Autodesk Fusion 360 part; units mm, degrees
(part 5 of 5)
equation "d1182 = ( FootHeight ) + PanHeight - DeckThick"
equation "d1184 = ( BaseX + LeftRun + FaucetGap + RightRun - RightSideDepth ) + ( ( RightSideDepth ) - ( ( Wall + DeckClearance + RimBorder ) + ( ( RightSideDepth ) - 2 * ( Wall + DeckClearance + RimBorder ) ) ) )"
equation "d1185 = ( BaseY + Depth + ModuleGap ) + ( ( ( ( RightReach ) - ( 14 * SlotPitch + SlotWidth ) ) / 2 ) + ( 11 * SlotPitch ) )"
equation "d1186 = ( RightSideDepth ) - 2 * ( Wall + DeckClearance + RimBorder )"
equation "d1187 = SlotWidth"
equation "d1188 = DeckThick"
equation "d1190 = ( FootHeight ) + PanHeight - DeckThick"
equation "d1192 = ( BaseX + LeftRun + FaucetGap + RightRun - RightSideDepth ) + ( ( RightSideDepth ) - ( ( Wall + DeckClearance + RimBorder ) + ( ( RightSideDepth ) - 2 * ( Wall + DeckClearance + RimBorder ) ) ) )"
equation "d1193 = ( BaseY + Depth + ModuleGap ) + ( ( ( ( RightReach ) - ( 14 * SlotPitch + SlotWidth ) ) / 2 ) + ( 12 * SlotPitch ) )"
equation "d1194 = ( RightSideDepth ) - 2 * ( Wall + DeckClearance + RimBorder )"
equation "d1195 = SlotWidth"
equation "d1196 = DeckThick"
equation "d1198 = ( FootHeight ) + PanHeight - DeckThick"
equation "d1200 = ( BaseX + LeftRun + FaucetGap + RightRun - RightSideDepth ) + ( ( RightSideDepth ) - ( ( Wall + DeckClearance + RimBorder ) + ( ( RightSideDepth ) - 2 * ( Wall + DeckClearance + RimBorder ) ) ) )"
equation "d1201 = ( BaseY + Depth + ModuleGap ) + ( ( ( ( RightReach ) - ( 14 * SlotPitch + SlotWidth ) ) / 2 ) + ( 13 * SlotPitch ) )"
equation "d1202 = ( RightSideDepth ) - 2 * ( Wall + DeckClearance + RimBorder )"
equation "d1203 = SlotWidth"
equation "d1204 = DeckThick"
equation "d1206 = ( FootHeight ) + PanHeight - DeckThick"
equation "d1208 = ( BaseX + LeftRun + FaucetGap + RightRun - RightSideDepth ) + ( ( RightSideDepth ) - ( ( Wall + DeckClearance + RimBorder ) + ( ( RightSideDepth ) - 2 * ( Wall + DeckClearance + RimBorder ) ) ) )"
equation "d1209 = ( BaseY + Depth + ModuleGap ) + ( ( ( ( RightReach ) - ( 14 * SlotPitch + SlotWidth ) ) / 2 ) + ( 14 * SlotPitch ) )"
equation "d1210 = ( RightSideDepth ) - 2 * ( Wall + DeckClearance + RimBorder )"
equation "d1211 = SlotWidth"
equation "d1212 = DeckThick"
equation "d1214 = ( FootHeight ) + PanHeight - DeckThick"
equation "d1216 = ( BaseX + LeftRun + FaucetGap + RightRun - RightSideDepth ) + ( ( RightSideDepth ) - ( ( ( RightSideDepth ) - Wall - DeckClearance - 4 mm ) + ( 5 mm ) ) )"
equation "d1217 = ( BaseY + Depth + ModuleGap ) + ( ( RightReach ) / 2 - 8 mm )"
equation "d1220 = DeckThick"
equation "d1222 = TouchChamfer"
equation "d1223 = FootHeight + PanHeight - DeckThick"
equation "d1225 = ( BaseX ) + ( ( Wall ) - DeckClearance )"
equation "d1226 = ( BaseY ) + ( 10 mm - DeckClearance )"
equation "d1227 = 2 mm + 2 * DeckClearance"
equation "d1228 = 5 mm + 2 * DeckClearance"
equation "d1229 = DeckThick"
equation "d1231 = FootHeight"
equation "d1233 = ( BaseX ) + ( Wall )"
equation "d1234 = ( BaseY ) + ( 10 mm )"
equation "d1237 = PanHeight"
equation "d1239 = FootHeight + PanHeight - DeckThick"
equation "d1241 = ( BaseX ) + ( ( ( TowerWidth ) - Wall - 2 mm ) - DeckClearance )"
equation "d1242 = ( BaseY ) + ( 10 mm - DeckClearance )"
equation "d1243 = 2 mm + 2 * DeckClearance"
equation "d1244 = 5 mm + 2 * DeckClearance"
equation "d1245 = DeckThick"
equation "d1247 = FootHeight"
equation "d1249 = ( BaseX ) + ( ( TowerWidth ) - Wall - 2 mm )"
equation "d1250 = ( BaseY ) + ( 10 mm )"
equation "d1253 = PanHeight"
equation "d1255 = FootHeight + PanHeight - DeckThick"
equation "d1257 = ( BaseX + TowerWidth + ModuleGap ) + ( ( Wall ) - DeckClearance )"
equation "d1258 = ( BaseY ) + ( 10 mm - DeckClearance )"
equation "d1259 = 2 mm + 2 * DeckClearance"
equation "d1260 = 5 mm + 2 * DeckClearance"
equation "d1261 = DeckThick"
equation "d1263 = FootHeight"
equation "d1265 = ( BaseX + TowerWidth + ModuleGap ) + ( Wall )"
equation "d1266 = ( BaseY ) + ( 10 mm )"
equation "d1269 = PanHeight"
equation "d1271 = FootHeight + PanHeight - DeckThick"
equation "d1273 = ( BaseX + TowerWidth + ModuleGap ) + ( ( ( LeftRun - TowerWidth - ModuleGap ) - Wall - 2 mm ) - DeckClearance )"
equation "d1274 = ( BaseY ) + ( 10 mm - DeckClearance )"
equation "d1275 = 2 mm + 2 * DeckClearance"
equation "d1276 = 5 mm + 2 * DeckClearance"
equation "d1277 = DeckThick"
equation "d1279 = FootHeight"
equation "d1281 = ( BaseX + TowerWidth + ModuleGap ) + ( ( LeftRun - TowerWidth - ModuleGap ) - Wall - 2 mm )"
equation "d1282 = ( BaseY ) + ( 10 mm )"
equation "d1285 = PanHeight"
equation "d1287 = FootHeight + PanHeight - DeckThick"
equation "d1289 = ( BaseX + LeftRun + FaucetGap ) + ( ( Wall ) - DeckClearance )"
equation "d1290 = ( BaseY ) + ( 10 mm - DeckClearance )"
equation "d1291 = 2 mm + 2 * DeckClearance"
equation "d1292 = 5 mm + 2 * DeckClearance"
equation "d1293 = DeckThick"
equation "d1295 = FootHeight"
equation "d1297 = ( BaseX + LeftRun + FaucetGap ) + ( Wall )"
equation "d1298 = ( BaseY ) + ( 10 mm )"
equation "d1301 = PanHeight"
equation "d1303 = FootHeight + PanHeight - DeckThick"
equation "d1305 = ( BaseX + LeftRun + FaucetGap ) + ( ( ( ( RightRun - ModuleGap ) / 2 ) - Wall - 2 mm ) - DeckClearance )"
equation "d1306 = ( BaseY ) + ( 10 mm - DeckClearance )"
equation "d1307 = 2 mm + 2 * DeckClearance"
equation "d1308 = 5 mm + 2 * DeckClearance"
equation "d1309 = DeckThick"
equation "d1311 = FootHeight"
equation "d1313 = ( BaseX + LeftRun + FaucetGap ) + ( ( ( RightRun - ModuleGap ) / 2 ) - Wall - 2 mm )"
equation "d1314 = ( BaseY ) + ( 10 mm )"
equation "d1317 = PanHeight"
equation "d1319 = FootHeight + PanHeight - DeckThick"
equation "d1321 = ( BaseX + LeftRun + FaucetGap + ( RightRun + ModuleGap ) / 2 ) + ( ( Wall ) - DeckClearance )"
equation "d1322 = ( BaseY ) + ( 10 mm - DeckClearance )"
equation "d1323 = 2 mm + 2 * DeckClearance"
equation "d1324 = 5 mm + 2 * DeckClearance"
equation "d1325 = DeckThick"
equation "d1327 = FootHeight"
equation "d1329 = ( BaseX + LeftRun + FaucetGap + ( RightRun + ModuleGap ) / 2 ) + ( Wall )"
equation "d1330 = ( BaseY ) + ( 10 mm )"
equation "d1333 = PanHeight"
equation "d1335 = FootHeight + PanHeight - DeckThick"
equation "d1337 = ( BaseX + LeftRun + FaucetGap + ( RightRun + ModuleGap ) / 2 ) + ( ( ( ( RightRun - ModuleGap ) / 2 ) - Wall - 2 mm ) - DeckClearance )"
equation "d1338 = ( BaseY ) + ( 10 mm - DeckClearance )"
equation "d1339 = 2 mm + 2 * DeckClearance"
equation "d1340 = 5 mm + 2 * DeckClearance"
equation "d1341 = DeckThick"
equation "d1343 = FootHeight"
equation "d1345 = ( BaseX + LeftRun + FaucetGap + ( RightRun + ModuleGap ) / 2 ) + ( ( ( RightRun - ModuleGap ) / 2 ) - Wall - 2 mm )"
equation "d1346 = ( BaseY ) + ( 10 mm )"
equation "d1349 = PanHeight"
equation "d1351 = FootHeight + PanHeight - DeckThick"
equation "d1353 = ( BaseX ) + ( 10 mm - DeckClearance )"
equation "d1354 = ( BaseY + Depth + ModuleGap ) + ( ( LeftReach ) - ( ( ( Wall ) - DeckClearance ) + ( 2 mm + 2 * DeckClearance ) ) )"
equation "d1355 = 5 mm + 2 * DeckClearance"
equation "d1356 = 2 mm + 2 * DeckClearance"
equation "d1357 = DeckThick"
equation "d1359 = FootHeight"
equation "d1361 = ( BaseX ) + ( 10 mm )"
equation "d1362 = ( BaseY + Depth + ModuleGap ) + ( ( LeftReach ) - ( ( Wall ) + ( 2 mm ) ) )"
equation "d1365 = PanHeight"
equation "d1367 = FootHeight + PanHeight - DeckThick"
equation "d1369 = ( BaseX ) + ( 10 mm - DeckClearance )"
equation "d1370 = ( BaseY + Depth + ModuleGap ) + ( ( LeftReach ) - ( ( ( ( LeftReach ) - Wall - 2 mm ) - DeckClearance ) + ( 2 mm + 2 * DeckClearance ) ) )"
equation "d1371 = 5 mm + 2 * DeckClearance"
equation "d1372 = 2 mm + 2 * DeckClearance"
equation "d1373 = DeckThick"
equation "d1375 = FootHeight"
equation "d1377 = ( BaseX ) + ( 10 mm )"
equation "d1378 = ( BaseY + Depth + ModuleGap ) + ( ( LeftReach ) - ( ( ( LeftReach ) - Wall - 2 mm ) + ( 2 mm ) ) )"
equation "d1381 = PanHeight"
equation "d1383 = FootHeight + PanHeight - DeckThick"
equation "d1385 = ( BaseX + LeftRun + FaucetGap + RightRun - RightSideDepth ) + ( ( RightSideDepth ) - ( ( 10 mm - DeckClearance ) + ( 5 mm + 2 * DeckClearance ) ) )"
equation "d1386 = ( BaseY + Depth + ModuleGap ) + ( ( Wall ) - DeckClearance )"
equation "d1387 = 5 mm + 2 * DeckClearance"
equation "d1388 = 2 mm + 2 * DeckClearance"
equation "d1389 = DeckThick"
equation "d1391 = FootHeight"
equation "d1393 = ( BaseX + LeftRun + FaucetGap + RightRun - RightSideDepth ) + ( ( RightSideDepth ) - ( ( 10 mm ) + ( 5 mm ) ) )"
equation "d1394 = ( BaseY + Depth + ModuleGap ) + ( Wall )"
equation "d1397 = PanHeight"
equation "d1399 = FootHeight + PanHeight - DeckThick"
equation "d1401 = ( BaseX + LeftRun + FaucetGap + RightRun - RightSideDepth ) + ( ( RightSideDepth ) - ( ( 10 mm - DeckClearance ) + ( 5 mm + 2 * DeckClearance ) ) )"
equation "d1402 = ( BaseY + Depth + ModuleGap ) + ( ( ( RightReach ) - Wall - 2 mm ) - DeckClearance )"
equation "d1403 = 5 mm + 2 * DeckClearance"
equation "d1404 = 2 mm + 2 * DeckClearance"
equation "d1405 = DeckThick"
equation "d1407 = FootHeight"
equation "d1409 = ( BaseX + LeftRun + FaucetGap + RightRun - RightSideDepth ) + ( ( RightSideDepth ) - ( ( 10 mm ) + ( 5 mm ) ) )"
equation "d1410 = ( BaseY + Depth + ModuleGap ) + ( ( RightReach ) - Wall - 2 mm )"
equation "d1413 = PanHeight"
named bodies: "R1_Integrated", "R1_RemovableGrate", "L1_Integrated", "L1_RemovableGrate", "L2_Integrated", "L2_RemovableGrate", "R2_Integrated", "R2_RemovableGrate", "LS_Integrated", "LS_RemovableGrate", "RS_Integrated", "RS_RemovableGrate"
